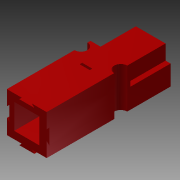
# Autodesk Inventor part: PowerPole45
Saved by Autodesk Inventor 2014 SP1 (Build 180222100, 222)
## iProperties
Created: 2016-03-18
Part Number: PowerPole45
Material: ABS Plastic
Document SubType Name: Modeling
Designer: Tyler
Density: 1.06 g/cm^3
Appearance: Smooth - Red
Author: Tyler
Autodesk Inventor part; units mm, degrees
ref_plane "YZ Plane" through (0, 0, 0) normal (1, 0, 0) x (0, 1, 0)
ref_plane "XZ Plane" through (0, 0, 0) normal (0, 1, 0) x (-1, 0, 0)
ref_plane "XY Plane" through (0, 0, 0) normal (0, 0, 1) x (1, 0, 0)
sketch "Sketch1" plane through (0, 0, 0) normal (0, 1, 0) x (-1, 0, 0)
  line L0 (-3.95, -3.95) -> (3.95, -3.95)
  line L1 (3.95, -3.95) -> (3.95, 3.95)
  line L2 (3.95, 3.95) -> (-3.95, 3.95)
  line L3 (-3.95, 3.95) -> (-3.95, -3.95)
  line L4 (-3.95, -3.95) -> (3.95, 3.95) construction
  line L5 (3.95, -3.95) -> (-3.95, 3.95) construction
  point P0 (0, 0)
  dimension "d0" = 7.9
  dimension "d1" = 7.9
  constraints: 12 end point, 2 midpoint, 2 parallel, 1 horizontal, 1 perpendicular
  measures "d0" distance of L2.end L1.end
  measures "d1" distance of L1.end L0.end
extrude "Extrusion1" add sketch "Sketch1" along normal blind 24.6
sketch "Sketch2" plane through (-3.95, 0, 3.95) normal (0, 0, 1) x (1, 0, 0)
  line L0 (7.9, 0) -> (7.9, 24.6) projected
  line L1 (0, 24.6) -> (7.9, 24.6) projected
  line L2 (0, 0) -> (0, 24.6) projected
  circle A0 centre (0, 14.7) radius 1.3
  circle A1 centre (7.9, 14.7) radius 1.3
  point P0 (3.95, 0)
  dimension "d4" = 2.6
  dimension "d5" = 2.6
  dimension "d6" = 9.9
  dimension "d7" = 9.9
  constraints: 2 centre point, 2 point on line
  measures "d4" diameter of A0
  measures "d5" diameter of A1
  measures "d6" distance from line of A0.centre L1
  measures "d7" distance from line of A1.centre L1
extrude "Extrusion2" cut sketch "Sketch2" against normal through all
sketch "Sketch3" plane through (0, 0, 0) normal (0, -1, 0) x (1, 0, 0)
  line L0 (-2.5, -2.5) -> (2.5, -2.5)
  line L1 (2.5, -2.5) -> (2.5, 2.5)
  line L2 (2.5, 2.5) -> (-2.5, 2.5)
  line L3 (-2.5, 2.5) -> (-2.5, -2.5)
  line L4 (-2.5, -2.5) -> (2.5, 2.5) construction
  line L5 (2.5, -2.5) -> (-2.5, 2.5) construction
  point P0 (0, 0)
  dimension "d10" = 5
  dimension "d11" = 5
  constraints: 12 end point, 2 midpoint, 2 parallel, 1 horizontal, 1 perpendicular
  measures "d10" distance of L2.end L1.end
  measures "d11" distance of L1.end L0.end
extrude "Extrusion3" cut sketch "Sketch3" against normal blind 15
sketch "Sketch4" plane through (0, 24.6, 0) normal (0, 1, 0) x (1, 0, 0)
  line L0 (-3.95, 3.95) -> (-3.95, -3.95) projected
  line L1 (-3.95, -3.95) -> (3.95, -3.95) projected
  line L2 (3.95, -3.95) -> (3.95, 3.95) projected
  line L3 (-3.95, 0) -> (-2.95, 0)
  line L4 (-2.95, 0) -> (-2.95, -2.95)
  line L5 (-2.95, -2.95) -> (2.95, -2.95)
  line L6 (2.95, -2.95) -> (2.95, 0)
  line L7 (2.95, 0) -> (3.95, 0)
  point P0 (0, 0)
  dimension "d14" = 1
  dimension "d15" = 1
  dimension "d16" = 1
  constraints: 10 end point, 2 midpoint, 2 parallel, 2 perpendicular, 1 collinear
  measures "d14" distance between parallel lines of L0 L4
  measures "d15" distance between parallel lines of L1 L5
  measures "d16" distance between parallel lines of L2 L6
extrude "Extrusion4" cut sketch "Sketch4" against normal blind 8
sketch "Sketch5" plane through (0, 24.6, 0) normal (0, 1, 0) x (1, 0, 0)
  line L0 (3.95, 3.95) -> (-3.95, 3.95) projected
  line L1 (-3.95, 3.95) -> (-3.95, 0) projected
  line L2 (-2.95, 2.95) -> (2.95, 2.95)
  line L3 (2.95, 2.95) -> (2.95, 0)
  line L4 (2.95, 0) -> (-2.95, 0)
  line L5 (-2.95, 0) -> (-2.95, 2.95)
  line L6 (-2.95, 2.95) -> (2.95, 0) construction
  line L7 (2.95, 2.95) -> (-2.95, 0) construction
  point P0 (0, 0)
  point P1 (0, 1.475)
  dimension "d19" = 1
  dimension "d20" = 1
  constraints: 12 end point, 2 midpoint, 2 parallel, 1 horizontal, 1 perpendicular
  measures "d19" distance between parallel lines of L0 L2
  measures "d20" distance between parallel lines of L1 L5
extrude "Extrusion5" cut sketch "Sketch5" against normal blind 8
sketch "Sketch6" plane through (0, 0, 0) normal (0, -1, 0) x (1, 0, 0)
  line L0 (3.95, -3.95) -> (-3.95, -3.95) projected
  line L1 (3.95, 3.95) -> (3.95, -3.95) projected
  line L2 (-3.95, -3.95) -> (-3.95, 3.95) projected
  line L3 (1.5, -4.45) -> (-1.5, -4.45)
  line L4 (1.5, -4.45) -> (1, -3.95)
  line L5 (-1.5, -4.45) -> (-1, -3.95)
  line L6 (3.95, -3.95) -> (2.5, -2.5) construction
  line L7 (4.45, -1.5) -> (4.45, 1.5)
  line L8 (4.45, -1.5) -> (3.95, -1)
  line L9 (4.45, 1.5) -> (3.95, 1)
  line L10 (3.95, 1) -> (3.95, -1)
  point P0 (0, 0)
  dimension "d23" = 3
  dimension "d24" = 1.5
  dimension "d26" = 0.5
  dimension "d27" = 45
  dimension "d28" = 45
  constraints: 16 end point, 4 point on line, 4 symmetric about line, 1 perpendicular
  measures "d23" distance of L3.start L3.end
  measures "d24" horizontal distance of point (0, 0) L3.end
  measures "d26" distance between parallel lines of L0 L3
  measures "d27" angle of L4 L3
  measures "d28" angle of L5 L3
extrude "Extrusion6" add sketch "Sketch6" against normal blind 12
sketch "Sketch7" plane through (0, 0, 0) normal (0, -1, 0) x (1, 0, 0)
  line L0 (-2.5, -2.5) -> (-2.5, 2.5) projected
  line L1 (-3.95, -3.95) -> (-3.95, 3.95) projected
  line L2 (-1.5, -4.45) -> (1.5, -4.45) projected
  line L3 (1.5, -4.45) -> (1, -3.95) projected
  line L4 (-3.95, -1) -> (-3.45, -1.5)
  line L5 (-3.45, -1.5) -> (-3.45, 1.5)
  line L6 (-3.45, 1.5) -> (-3.95, 1)
  line L7 (-3.95, 1) -> (-3.95, -1)
  line L8 (-3.95, 3.95) -> (-2.5, 2.5) construction
  line L9 (1, 3.95) -> (1.5, 3.45)
  line L10 (1.5, 3.45) -> (-1.5, 3.45)
  line L11 (-1.5, 3.45) -> (-1, 3.95)
  line L12 (-1, 3.95) -> (1, 3.95)
  point P0 (0, 0)
  dimension "d34" = 3
  dimension "d35" = 1.5
  dimension "d36" = 0.5
  constraints: 18 end point, 4 symmetric about line, 3 perpendicular, 3 point on line, 2 parallel
  measures "d34" distance of L4.end L5.end
  measures "d35" vertical distance of point (0, 0) L5.end
  measures "d36" distance between parallel lines of L1 L5
extrude "Extrusion7" cut sketch "Sketch7" against normal blind 12
body "Solid1"
